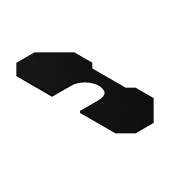
# Autodesk Inventor part: BackPlateBottom
Saved by Autodesk Inventor 2014 (Build 180170000, 170)
## iProperties
Created: 2014-08-10
Part Number: BackPlateBottom
Material: Generic
Document SubType Name: Modeling
Designer: Peele
Density: 1 g/cm^3
Appearance: Glossy - Black
Author: Peele
Autodesk Inventor part; units mm, degrees
ref_plane "YZ Plane" through (0, 0, 0) normal (1, 0, 0) x (0, 1, 0)
ref_plane "XZ Plane" through (0, 0, 0) normal (0, 1, 0) x (-1, 0, 0)
ref_plane "XY Plane" through (0, 0, 0) normal (0, 0, 1) x (1, 0, 0)
sketch "Sketch1" plane through (0, 0, 0) normal (0, 0, 1) x (1, 0, 0)
  line L0 (-125, -48) -> (125, -48)
  line L1 (125, -48) -> (125, 48)
  line L2 (125, 48) -> (-125, 48)
  line L3 (-125, 48) -> (-125, -48)
  line L4 (-125, -48) -> (125, 48) construction
  line L5 (125, -48) -> (-125, 48) construction
  point P0 (0, 0)
  dimension "d0" = 250
  dimension "d1" = 96
  constraints: 12 end point, 2 midpoint, 2 parallel, 1 horizontal, 1 perpendicular
  measures "d0" distance of L1.end L2.end
  measures "d1" distance of L0.end L1.end
extrude "Extrusion1" add sketch "Sketch1" along normal blind 4
sketch "Sketch2" plane through (0, 0, 4) normal (0, 0, 1) x (1, 0, 0)
  line L0 (125, -48) -> (125, 48) projected
  line L1 (125, 48) -> (-125, 48) projected
  line L2 (-125, 48) -> (-125, -48) projected
  line L3 (-125, 48) -> (-150, 23)
  line L4 (-150, 23) -> (-150, -23)
  line L5 (-150, -23) -> (-125, -48)
  line L6 (125, 48) -> (150, 23)
  line L7 (150, 23) -> (150, -23)
  line L8 (150, -23) -> (125, -48)
  line L9 (-125, 48) -> (-100, 73)
  line L10 (-100, 73) -> (-55, 73)
  line L11 (-55, 73) -> (-30, 48)
  line L12 (-125, -48) -> (-30, 48)
  line L13 (125, 48) -> (100, 73)
  line L14 (100, 73) -> (55, 73)
  line L15 (55, 73) -> (30, 48)
  line L16 (125, -48) -> (30, 48)
  circle A0 centre (-137.5, 15.5) radius 2
  circle A1 centre (-137.5, -14.5) radius 2
  circle A2 centre (-92.5, 60.5) radius 2
  circle A3 centre (-62.5, 60.5) radius 2
  circle A4 centre (62.5, 60.5) radius 2
  circle A5 centre (92.5, 60.5) radius 2
  circle A6 centre (137.5, 15.5) radius 2
  circle A7 centre (137.5, -14.5) radius 2
  point P0 (0, 0)
  dimension "d4" = 25
  dimension "d5" = 45
  dimension "d6" = 30
  dimension "d7" = 30
  dimension "d9" = 7.5
  dimension "d10" = 12.5
  dimension "d11" = 4
  dimension "d12" = 30
  dimension "d13" = 7.5
  dimension "d14" = 7.5
  dimension "d15" = 7.5
  dimension "d16" = 12.5
  dimension "d17" = 12.5
  constraints: 28 end point, 8 centre point, 8 equal length, 7 equal radius, 4 horizontal alignment, 3 collinear, 3 parallel, 2 perpendicular, 2 point on line, 2 vertical alignment
  measures "d4" distance between parallel lines of L10 L1
  measures "d5" distance of L9.end L10.end
  measures "d6" distance of A2.centre A3.centre
  measures "d7" distance of A1.centre A0.centre
  measures "d9" horizontal distance of A2.centre L9.end
  measures "d10" distance from line of A3.centre L1
  measures "d11" diameter of A3
  measures "d12" distance of A5.centre A4.centre
  measures "d13" horizontal distance of A5.centre L13.end
  measures "d14" vertical distance of L3.end A0.centre
  measures "d15" vertical distance of L6.end A6.centre
  measures "d16" distance from line of A0.centre L2
  measures "d17" distance from line of A6.centre L0
extrude "Extrusion2" add sketch "Sketch2" against normal blind 4 contours L0 L6 L7 L8 | L1 L15 L14 L13 | L1 L9 L10 L11 | L2 L5 L4 L3
sketch "Sketch3" plane through (0, 0, 4) normal (0, 0, 1) x (1, 0, 0)
  line L0 (-125, -48) -> (125, -48) projected
  circle A0 centre (0, 0) radius 35
  line L1 (-35, 0) -> (-35, -48)
  line L2 (-35, -48) -> (35, -48)
  line L3 (35, -48) -> (35, 0)
  dimension "d20" = 70
  constraints: 6 end point, 2 point on circle, 2 point on line, 2 tangent, 1 centre point, 1 coincident, 1 perpendicular, 1 vertical
  measures "d20" diameter of A0
extrude "Extrusion3" cut sketch "Sketch3" against normal blind 4
sketch "Sketch4" plane through (0, 0, 4) normal (0, 0, 1) x (1, 0, 0)
  line L0 (55, 73) -> (30, 48) projected
  line L1 (30, 48) -> (-30, 48) projected
  line L2 (-30, 48) -> (-55, 73) projected
  line L3 (-42.5, 60.5) -> (42.5, 60.5)
  line L4 (42.5, 60.5) -> (42.5, 48)
  line L5 (42.5, 48) -> (-42.5, 48)
  line L6 (-42.5, 48) -> (-42.5, 60.5)
  constraints: 8 end point, 2 midpoint, 2 parallel, 1 collinear, 1 horizontal, 1 perpendicular
extrude "Extrusion4" add sketch "Sketch4" against normal blind 4 contours L0 L1 L2 L3
equation "\"d7\" = d6"
equation "\"d9\" = -0.5 * d6 + 0.5 * d5"
equation "\"d12\" = d6"
equation "\"d13\" = d9"
equation "\"d14\" = d9"
equation "\"d15\" = d13"
body "Solid1"
